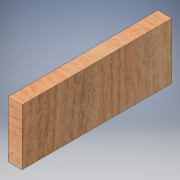
# Autodesk Inventor part: sidePlate
Saved by Autodesk Inventor 2016 (Build 200138000, 138)
## iProperties
Created: 2015-09-21
Part Number: sidePlate
Material: Generic
Document SubType Name: Modeling
Designer: xdlea
Density: 1 g/cm^3
Appearance: Birch - Natural Polished
Height: 3.000 in
Author: xdlea
Autodesk Inventor part; units mm, degrees
ref_plane "YZ Plane" through (0, 0, 0) normal (1, 0, 0) x (0, 1, 0)
ref_plane "XZ Plane" through (0, 0, 0) normal (0, 1, 0) x (-1, 0, 0)
ref_plane "XY Plane" through (0, 0, 0) normal (0, 0, 1) x (1, 0, 0)
sketch "Sketch1" plane through (0, 0, 0) normal (1, 0, 0) x (0, 1, 0)
  line L0 (-38.1, 101.6) -> (38.1, 101.6)
  line L1 (38.1, 101.6) -> (38.1, -101.6)
  line L2 (38.1, -101.6) -> (-38.1, -101.6)
  line L3 (-38.1, -101.6) -> (-38.1, 101.6)
  line L4 (-38.1, 101.6) -> (38.1, -101.6) construction
  line L5 (38.1, 101.6) -> (-38.1, -101.6) construction
  point P0 (0, 0)
  dimension "d0" = 203.2
  dimension "d1" = 76.2
  constraints: 12 end point, 2 midpoint, 2 parallel, 1 horizontal, 1 perpendicular
  measures "d0" distance of L0.end L1.end
  measures "d1" distance of L1.end L2.end
extrude "Extrusion1" add sketch "Sketch1" along normal blind 19.05
equation "\"d0\" = Width"
equation "\"d1\" = Height"
equation "\"d2\" = Thickness"
equation "\"Height\" = 76.2"
equation "\"Width\" = 203.2"
equation "\"Thickness\" = 19.05"
body "Solid1"
